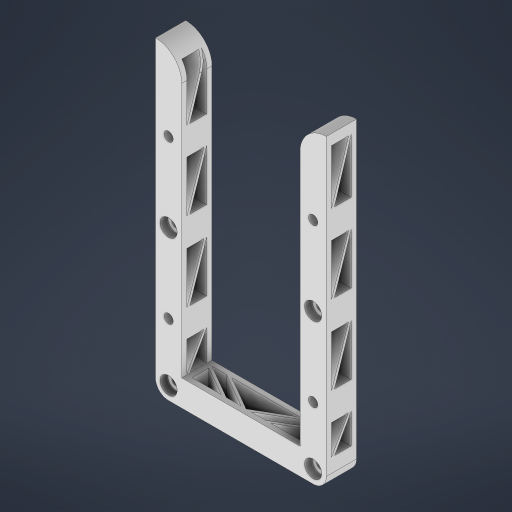
# Autodesk Inventor part: middle spacer top
Saved by Autodesk Inventor 2023 (Build 270158000, 158)
## iProperties
Created: 2022-05-31
Part Number: middle spacer top
Material: Generic
Document SubType Name: Modeling
Designer: vibhu
Density: 1 g/cm^3
Appearance: Default
Author: vibhu
Autodesk Inventor part; units mm, degrees
ref_plane "YZ Plane" through (0, 0, 0) normal (1, 0, 0) x (0, 1, 0)
ref_plane "Work Plane1" through (0, 0, 0) normal (0, 0, 1) x (1, 0, 0)
ref_plane "Work Plane2" through (-68.4987, -48.7487, 11.5) normal (0, 0, 1) x (0.7071068, -0.7071068, 0)
sketch "Sketch1" plane through (0, 0, 0) normal (0, 0, 1) x (1, 0, 0)
  circle A0 centre (43.75, 66) radius 1.75 projected
  circle A1 centre (-11.25, 6) radius 1.75 projected
  circle A2 centre (-11.25, 66) radius 1.75 projected
  circle A3 centre (43.75, 6) radius 1.75 projected
  circle A4 centre (-11.25, -16) radius 1.75 projected
  circle A5 centre (-11.25, 36) radius 1.75 projected
  circle A6 centre (43.75, -16) radius 1.75 projected
  circle A7 centre (43.75, 36) radius 1.75 projected
  line L0 (-12.875, 48.1854) -> (-9.625, 48.1854) projected
  line L1 (-14.5, 51) -> (-12.875, 48.1854) projected
  line L2 (-12.875, 53.8146) -> (-14.5, 51) projected
  line L3 (-9.625, 53.8146) -> (-12.875, 53.8146) projected
  line L4 (-8, 51) -> (-9.625, 53.8146) projected
  line L5 (-9.625, 48.1854) -> (-8, 51) projected
  line L6 (-12.875, 18.1854) -> (-9.625, 18.1854) projected
  line L7 (-14.5, 21) -> (-12.875, 18.1854) projected
  line L8 (-12.875, 23.8146) -> (-14.5, 21) projected
  line L9 (-9.625, 23.8146) -> (-12.875, 23.8146) projected
  line L10 (-8, 21) -> (-9.625, 23.8146) projected
  line L11 (-9.625, 18.1854) -> (-8, 21) projected
  line L12 (42.125, 48.1854) -> (45.375, 48.1854) projected
  line L13 (40.5, 51) -> (42.125, 48.1854) projected
  line L14 (42.125, 53.8146) -> (40.5, 51) projected
  line L15 (45.375, 53.8146) -> (42.125, 53.8146) projected
  line L16 (47, 51) -> (45.375, 53.8146) projected
  line L17 (45.375, 48.1854) -> (47, 51) projected
  line L18 (42.125, 18.1854) -> (45.375, 18.1854) projected
  line L19 (40.5, 21) -> (42.125, 18.1854) projected
  line L20 (42.125, 23.8146) -> (40.5, 21) projected
  line L21 (45.375, 23.8146) -> (42.125, 23.8146) projected
  line L22 (47, 21) -> (45.375, 23.8146) projected
  line L23 (45.375, 18.1854) -> (47, 21) projected
  line L24 (14.625, -18.8146) -> (17.875, -18.8146) projected
  line L25 (13, -16) -> (14.625, -18.8146) projected
  line L26 (14.625, -13.1854) -> (13, -16) projected
  line L27 (17.875, -13.1854) -> (14.625, -13.1854) projected
  line L28 (19.5, -16) -> (17.875, -13.1854) projected
  line L29 (17.875, -18.8146) -> (19.5, -16) projected
  arc A8 (43.75, -21) -> (48.75, -16) centre (43.75, -16) ccw projected
  line L30 (48.75, -16) -> (48.75, 96) projected
  arc A9 (48.75, 96) -> (38.75, 86) centre (48.75, 86) ccw projected
  line L31 (38.75, 86) -> (38.75, 51) projected
  line L32 (38.75, 51) -> (38.75, -11) projected
  line L33 (38.75, -11) -> (-6.25, -11) projected
  line L34 (-6.25, -11) -> (-6.25, 51) projected
  line L35 (-6.25, 51) -> (-6.25, 86) projected
  arc A10 (-6.25, 86) -> (-16.25, 96) centre (-16.25, 86) ccw projected
  line L36 (-16.25, 96) -> (-16.25, -16) projected
  arc A11 (-16.25, -16) -> (-11.25, -21) centre (-11.25, -16) ccw projected
  line L37 (-11.25, -21) -> (43.75, -21) projected
  circle A12 centre (43.75, 51) radius 1.75
  circle A13 centre (-11.25, 51) radius 1.75
  circle A14 centre (-11.25, 21) radius 1.75
  circle A15 centre (43.75, 21) radius 1.75
  circle A16 centre (16.25, -16) radius 1.75 projected
  point P0 (0, 0)
  constraints: 4 centre point, 8 other
extrude "Extrusion1" add sketch "Sketch1" along normal up to surface (11.5 mm away) contours L1 L2 L3 L4 L5 L0 | L7 L8 L9 L10 L11 L6 | L13 L14 L15 L16 L17 L12 | L19 L20 L21 L22 L23 L18 | L25 L26 L27 L28 L29 L24 | L37 A11 L36 A10 L35 L34 L33 L32 L31 A9 L30 A8 | A12 | A13 | A14 | A15 | A16
sketch "Sketch2" plane through (-11.25, -21, 11.5) normal (0, 0, 1) x (1, 0, 0)
  circle A0 centre (0, 5) radius 1.75 construction
  circle A1 centre (0, 57) radius 1.75 construction
  circle A2 centre (55, 57) radius 1.75 construction
  circle A3 centre (55, 5) radius 1.75 construction
  circle A4 centre (0, 5) radius 1.75 projected
  circle A5 centre (0, 5) radius 3.25
  circle A6 centre (55, 5) radius 1.75 projected
  circle A7 centre (55, 5) radius 3.25
  circle A8 centre (55, 57) radius 3.25
  circle A9 centre (0, 57) radius 3.25
  point P0 (11.25, 21)
  dimension "d2" = 6.5
  constraints: 4 centre point, 4 coincident, 3 equal radius
  measures "d2" diameter of A5
extrude "Spacer Join Countersink" cut sketch "Sketch2" against normal blind 3 draft 2 contours A4 | A5 | A6 | A7 | A8 | A9
sketch "Sketch3" plane through (0, 0, 0) normal (0, 0, -1) x (-1, 0, 0)
  circle A0 centre (-43.75, 66) radius 1.75 construction
  circle A1 centre (11.25, 66) radius 1.75 construction
  circle A2 centre (11.25, 6) radius 1.75 construction
  circle A3 centre (-43.75, 6) radius 1.75 construction
  circle A4 centre (-43.75, 66) radius 3.25 construction
  circle A5 centre (11.25, 66) radius 1.75 projected
  circle A6 centre (11.25, 66) radius 3.25 construction
  circle A7 centre (11.25, 6) radius 1.75 projected
  circle A8 centre (11.25, 6) radius 3.25 construction
  circle A9 centre (-43.75, 6) radius 1.75 projected
  circle A10 centre (-43.75, 6) radius 3.25 construction
  line L0 (8.4354, 64.375) -> (8.4354, 67.625)
  line L1 (8.4354, 7.625) -> (8.4354, 4.375)
  line L2 (-41.2226, 8.0433) -> (-43.75, 9.25)
  line L3 (-43.75, 9.25) -> (-46.5646, 7.625)
  line L4 (-46.5646, 7.625) -> (-46.5646, 4.375)
  line L5 (-46.5646, 4.375) -> (-43.75, 2.75)
  line L6 (-43.75, 2.75) -> (-40.9354, 4.375)
  line L7 (-40.9354, 4.375) -> (-40.9354, 7.625)
  line L8 (-40.9354, 7.625) -> (-43.75, 9.25)
  line L9 (8.4354, 4.375) -> (11.25, 2.75)
  line L10 (11.25, 2.75) -> (14.0646, 4.375)
  line L11 (14.0646, 4.375) -> (14.0646, 7.625)
  line L12 (14.0646, 7.625) -> (11.25, 9.25)
  line L13 (11.25, 9.25) -> (8.4354, 7.625)
  line L14 (-46.5646, 67.625) -> (-46.5646, 64.375)
  line L15 (-46.5646, 64.375) -> (-43.75, 62.75)
  line L16 (-43.75, 62.75) -> (-40.9354, 64.375)
  line L17 (-40.9354, 64.375) -> (-40.9354, 67.625)
  line L18 (-40.9354, 67.625) -> (-43.75, 69.25)
  line L19 (-43.75, 69.25) -> (-46.5646, 67.625)
  line L20 (11.25, 62.75) -> (8.4354, 64.375)
  line L21 (14.0646, 64.375) -> (11.25, 62.75)
  line L22 (14.0646, 67.625) -> (14.0646, 64.375)
  line L23 (11.25, 69.25) -> (14.0646, 67.625)
  line L24 (8.4354, 67.625) -> (11.25, 69.25)
  point P0 (0, 0)
  dimension "d7" = 360
  dimension "d9" = 6.5
  dimension "d20" = 360
  dimension "d24" = 360
  dimension "d28" = 360
  constraints: 50 end point, 8 coincident, 8 point on circle, 4 centre point, 4 vertical, 3 equal radius, 76 other
  measures "d9" diameter of A10
extrude "nut holes" cut sketch "Sketch3" against normal blind 5
sketch "Sketch4" plane through (-16.25, -16, 0) normal (-1, 0, 0) x (0, 0, 1)
  line L0 (9.5, 87.25) -> (2, 87.25)
  line L1 (2, 87.25) -> (2, 108)
  line L2 (2, 108) -> (9.5, 108)
  line L3 (9.5, 108) -> (9.5, 87.25)
  line L4 (0, 112) -> (11.5, 112) projected
  line L5 (11.5, 0) -> (11.5, 112) projected
  line L6 (0, 112) -> (0, 0) projected
  line L7 (11.5, 80.25) -> (11.5, 83.75) projected
  line L8 (9.5, 76.75) -> (2, 76.75)
  line L9 (2, 76.75) -> (2, 57.3548)
  line L10 (2, 57.3548) -> (9.5, 57.3548)
  line L11 (9.5, 57.3548) -> (9.5, 76.75)
  line L12 (8.5, 50.25) -> (8.5, 53.75) projected
  line L13 (0, 53.75) -> (0, 50.25) projected
  line L14 (0, 1.75) -> (0, -1.75) projected
  line L15 (9.5, 46.6452) -> (2, 46.6452)
  line L16 (2, 46.6452) -> (2, 27.25)
  line L17 (2, 27.25) -> (9.5, 27.25)
  line L18 (9.5, 27.25) -> (9.5, 46.6452)
  line L19 (8.5, 48.6452) -> (8.5, 55.3548) projected
  line L20 (11.5, 55.25) -> (11.5, 48.75) projected
  line L21 (8.5, -3.3548) -> (8.5, 3.3548) projected
  line L22 (11.5, 3.25) -> (11.5, -3.25) projected
  line L23 (9.5, 16.75) -> (2, 16.75)
  line L24 (2, 16.75) -> (2, 5.3548)
  line L25 (2, 5.3548) -> (9.5, 5.3548)
  line L26 (9.5, 5.3548) -> (9.5, 16.75)
  line L27 (9.5, 87.25) -> (3.0472, 108)
  line L28 (2, 108) -> (8.4528, 87.25)
  line L29 (3.0538, 76.75) -> (9.5, 57.3548)
  line L30 (8.4462, 57.3548) -> (2, 76.75)
  line L31 (3.0538, 46.6452) -> (9.5, 27.25)
  line L32 (8.4462, 27.25) -> (2, 46.6452)
  line L33 (9.5, 5.3548) -> (3.145, 16.75)
  line L34 (2, 16.75) -> (8.355, 5.3548)
  point P0 (5.75, 108)
  point P1 (0, 85.25)
  point P2 (0, 78.75)
  point P3 (5.75, 87.25)
  point P4 (0, 25.25)
  point P5 (0, 18.75)
  dimension "d32" = 4
  dimension "d33" = 2
  dimension "d34" = 2
  dimension "d37" = 2
  dimension "d38" = 2
  dimension "d41" = 2
  dimension "d42" = 2
  dimension "d43" = 2
  dimension "d44" = 2
  dimension "d45" = 2
  dimension "d47" = 1
  dimension "d48" = 1
  dimension "d49" = 1
  dimension "d50" = 1
  constraints: 48 end point, 12 parallel, 8 point on line, 6 collinear, 4 horizontal, 4 perpendicular, 2 midpoint
  measures "d32" distance from line of point (5.75, 108) L4
  measures "d33" distance between parallel lines of L5 L3
  measures "d34" distance between parallel lines of L6 L1
  measures "d37" vertical distance of point (0, 85.25) point (5.75, 87.25)
  measures "d38" distance from line of L8 point (0, 78.75)
  measures "d41" distance from line of L19.end L10
  measures "d42" distance from line of L19.start L15
  measures "d43" distance from line of L17 point (0, 25.25)
  measures "d44" distance from line of L23 point (0, 18.75)
  measures "d45" distance from line of L21.end L25
  measures "d47" distance between parallel lines of L27 L28
  measures "d48" distance between parallel lines of L29 L30
  measures "d49" distance between parallel lines of L32 L31
  measures "d50" distance between parallel lines of L34 L33
extrude "Extrusion4" cut sketch "Sketch4" against normal blind 65 contours L27 L2 L3 | L0 L1 L28 | L11 L29 L8 | L30 L10 L9 | L18 L31 L15 | L32 L17 L16 | L26 L33 L23 | L34 L25 L24
sketch "Sketch5" plane through (-11.25, -21, 0) normal (0, -1, 0) x (1, 0, 0)
  line L0 (3.3548, 8.5) -> (-3.3548, 8.5) projected
  line L1 (-3.25, 11.5) -> (3.25, 11.5) projected
  line L2 (58.3548, 8.5) -> (51.6452, 8.5) projected
  line L3 (51.75, 11.5) -> (58.25, 11.5) projected
  line L4 (7, 9.5) -> (7, 3.1547)
  line L5 (7, 3.1547) -> (17.9904, 9.5)
  line L6 (17.9904, 9.5) -> (7, 9.5)
  line L7 (7, 2) -> (19.9904, 9.5)
  line L8 (19.9904, 9.5) -> (35.0096, 9.5)
  line L9 (0, 0) -> (55, 0) projected
  line L10 (35.0096, 9.5) -> (48, 2)
  line L11 (48, 2) -> (7, 2)
  line L12 (37.0096, 9.5) -> (48, 3.1547)
  line L13 (48, 3.1547) -> (48, 9.5)
  line L14 (48, 9.5) -> (37.0096, 9.5)
  line L15 (55, 11.5) -> (0, 11.5) projected
  line L16 (12.5096, 2) -> (25.5, 9.5)
  line L17 (14.5096, 2) -> (27.5, 9.5)
  line L18 (27.5, 9.5) -> (40.4904, 2)
  line L19 (29.5, 9.5) -> (42.4904, 2)
  line L20 (50, 0) -> (50, 11.5) projected
  line L21 (5, 0) -> (5, 11.5) projected
  point P0 (27.5, 11.5)
  dimension "d53" = 2
  dimension "d57" = 2
  dimension "d58" = 1
  dimension "d60" = 1
  dimension "d62" = 1
  dimension "d63" = 1
  dimension "d64" = 60
  dimension "d67" = 2
  dimension "d68" = 2
  constraints: 28 end point, 8 parallel, 6 point on line, 3 midpoint, 3 vertical alignment, 2 collinear, 1 coincident, 1 perpendicular, 1 vertical
  measures "d53" distance between parallel lines of L15 L14
  measures "d57" distance between parallel lines of L9 L11
  measures "d58" distance between parallel lines of L7 L5
  measures "d60" distance between parallel lines of L12 L10
  measures "d62" distance between parallel lines of L17 L16
  measures "d63" distance between parallel lines of L19 L18
  measures "d64" angle of L5 L4
  measures "d67" distance between parallel lines of L4 L21
  measures "d68" distance between parallel lines of L13 L20
extrude "Extrusion5" cut sketch "Sketch5" against normal up to surface (10 mm away) contours L6 L5 L4 | L7 L8 L16 L11 | L17 L18 L11 | L8 L10 L11 L19 | L14 L13 L12
body "Solid1"
